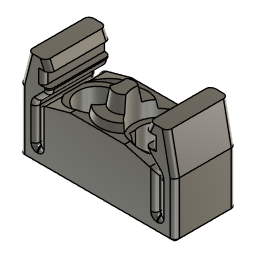
Lijn sensor lego adapter door Joep v9 (Autodesk Fusion 360 design; units mm, degrees)
Autodesk Fusion 360 part; units mm, degrees
note: some values were not read from the file. Chosen so that the rebuilt part matches the saved one: which face or edge a step refers to; which pieces of a blend or face edit are solid. Set by a fixed rule: which sketch regions a step uses.
sketch "Sketch1" plane through (0, 0, 0) normal (0, 1, 0) x (1, 0, 0)
  line L0 (41.5732, -34.0227) -> (56.5732, -34.0227)
  line L1 (41.5732, -34.0227) -> (41.5732, -28.0227)
  line L2 (41.5732, -28.0227) -> (41.0732, -28.0227)
  line L3 (42.0732, -35.2227) -> (42.0732, -37.0227)
  line L4 (42.0732, -37.0227) -> (42.8732, -37.0227)
  line L5 (42.8732, -37.0227) -> (42.3408, -38.2227)
  line L6 (42.3408, -38.2227) -> (39.0732, -38.2227)
  line L7 (49.0732, -34.0227) -> (49.0732, -26.0227) construction
  line L8 (42.8732, -34.6227) -> (41.0732, -32.8227)
  line L9 (41.0732, -32.8227) -> (41.0732, -28.0227)
  line L10 (39.0732, -26.0227) -> (39.0732, -38.2227)
  line L11 (55.2732, -37.0227) -> (55.8057, -38.2227)
  line L12 (56.0732, -37.0227) -> (55.2732, -37.0227)
  line L13 (56.0732, -35.2227) -> (56.0732, -37.0227)
  line L14 (55.8057, -38.2227) -> (59.0732, -38.2227)
  line L15 (59.0732, -26.0227) -> (39.0732, -26.0227)
  line L16 (59.0732, -26.0227) -> (59.0732, -38.2227)
  line L17 (57.0732, -32.8227) -> (57.0732, -28.0227)
  line L18 (56.5732, -28.0227) -> (57.0732, -28.0227)
  line L19 (56.5732, -34.0227) -> (56.5732, -28.0227)
  line L20 (42.0732, -35.2227) -> (42.8732, -35.2227)
  line L21 (42.8732, -35.2227) -> (42.8732, -34.6227)
  line L22 (56.0732, -35.2227) -> (55.2732, -35.2227)
  line L23 (55.2732, -35.2227) -> (55.2732, -34.6227)
  line L24 (55.2732, -34.6227) -> (57.0732, -32.8227)
  line L25 (41.0732, -28.0227) -> (39.0732, -28.0227)
  line L26 (57.0732, -28.0227) -> (59.0732, -28.0227)
  dimension "d3" = 3
  dimension "d5" = 1.2
  dimension "d6" = 0.8
  dimension "d15" = 1.8
  dimension "d16" = 0.5
  dimension "d17" = 2
  dimension "d18" = 14
  dimension "d19" = 8
  dimension "d20" = 15
  dimension "d21" = 20
  dimension "d67" = 0.6
  dimension "d68" = 0.8
  dimension "d85" = 45
  dimension "d86" = 2
  constraint horizontal L0
  constraint perpendicular L0 L1
  constraint perpendicular L1 L2
  constraint perpendicular L3 L4
  constraint horizontal L6
  constraint vertical L7
  constraint perpendicular L2 L9
  constraint coincident L6.end L10.end
  constraint symmetric L10.start L7 L15.start
  constraint symmetric L0.start L7 L0.end
  constraint symmetric L1.end L7 L18.start
  constraint symmetric L3.start L7 L13.start
  constraint symmetric L3.end L7 L12.start
  constraint symmetric L4.end L7 L11.start
  constraint symmetric L5.end L7 L11.end
  constraint symmetric L6.end L7 L14.end
  constraint symmetric L7 L2.end L17.end
  constraint symmetric L7 L8.end L17.start
  constraint symmetric L7 L6.end L14.end
  constraint coincident L0.end L19.start
  constraint coincident L10.start L15.end
  constraint midpoint L0 L7.start
  constraint midpoint L7.end L15
  constraint perpendicular L3 L20
  constraint perpendicular L20 L21
  constraint symmetric L7 L20.end L22.end
  constraint symmetric L7 L8.start L23.end
  constraint coincident L13.start L22.start
  constraint coincident L10 L25.end
  constraint perpendicular L10 L25
  constraint coincident L16 L26.end
  constraint perpendicular L16 L26
  constraint vertical L17
  measures "d3" distance of L0 L4
  measures "d5" distance of L4 L6
  measures "d6" distance of L3.end L4.end
  measures "d15" distance of L3.start L3.end
  measures "d16" distance of L1 L9
  measures "d17" distance of L9 L10
  measures "d18" distance of L3 L13
  measures "d19" distance of L0 L15
  measures "d20" distance of L1 L19
  measures "d21" distance of L10 L16
  measures "d67" distance of L20.end L8.start
  measures "d68" distance of L3.start L20.end
  measures "d85" angle of L8 L9
  measures "d86" distance of L2 L15
extrude "Extrude1" add sketch "Sketch1" along normal blind 7.9 contours L0 L1 L8 | L0 L1 L2 L8 L10 L15 L16 L18 L19 L24 L25 L26 | L0 L19 L24
sketch "Sketch2" plane through (0, 0, 26.0227) normal (0, 0, -1) x (1, 0, 0)
  circle A0 centre (45.0732, -3.95) radius 2.5
  circle A1 centre (53.0732, -3.95) radius 2.5
  line L0 (45.0732, -3.95) -> (53.0732, -3.95) construction
  line L1 (49.0732, 0) -> (49.0732, -7.9) construction
  circle A2 centre (49.0732, -3.45) radius 1.65
  circle A3 centre (49.0732, -3.45) radius 3
  line L2 (59.0732, 0) -> (39.0732, 0)
  line L3 (59.0732, -7.9) -> (39.0732, -7.9)
  circle A4 centre (53.0732, -3.95) radius 3.25
  circle A5 centre (45.0732, -3.95) radius 3.25
  dimension "d12" = 5
  dimension "d13" = 8
  dimension "d23" = 0.5
  dimension "d24" = 3.3
  dimension "d25" = 6
  dimension "d34" = 6.5
  constraint equal A0 A1
  constraint coincident A0.centre L0.start
  constraint coincident A1.centre L0.end
  constraint horizontal L0
  constraint midpoint L0 L1
  constraint midpoint L1.start L2
  constraint midpoint L1.end L3
  constraint concentric A1 A4
  constraint concentric A0 A5
  constraint equal A4 A5
  constraint coincident A2.centre A3.centre
  constraint coincident L1 A2.centre
  measures "d12" diameter of A0
  measures "d13" distance of A0.centre A1.centre
  measures "d23" distance of L0 A2.centre
  measures "d24" diameter of A2
  measures "d25" diameter of A3
  measures "d34" diameter of A4
extrude "Extrude3" add sketch "Sketch2" against normal blind 1 from surface at -8 contours A0 A2 | A0 A2 A5 | A0 A2 A3 | A0 A2 A3 A5 | A0 A2 A3 A5 | A2 A3 A4 A5 | A2 A4 A5 | A2 A3 A4 A5 | A1 A2 A3 A4 | A1 A2 A4 | A1 A2 A3 A4 | A1 A2 | A1 A2 A3
extrude "Extrude4" add sketch "Sketch2" against normal blind 2 draft -10 from surface at -9 contours A0 A2 | A0 A2 A5 | A2 A4 A5 | A1 A2 A4 | A1 A2
chamfer "Chamfer1" distance 0.2 distance2 1 1 edges at (46.2763, 4.5348, 34.0227) measured on face at (43.0732, 3.7833, 34.0227)
extrude "Extrude2" cut sketch "Sketch2" against normal blind 10.5 contours A0 A2 | A0 A2 A3 | A0 A3 | A1 A2 | A1 A2 A3 | A1 A3
extrude "Extrude5" cut sketch "Sketch2" against normal blind 1 contours A0 A2 | A0 A2 A5 | A0 A2 A3 | A0 A2 A3 A5 | A0 A2 A3 A5 | A0 A3 | A0 A3 A5 | A1 A2 A3 A4 | A1 A2 A4 | A1 A2 A3 A4 | A1 A3 A4 | A1 A2 | A1 A2 A3 | A1 A3
extrude "Extrude6" cut sketch "Sketch2" against normal blind 4 from surface at -7 contours A0 A2 | A0 A2 A5 | A0 A2 A3 | A0 A2 A3 A5 | A0 A2 A3 A5 | A0 A3 | A0 A3 A5 | A1 A2 A3 A4 | A1 A2 A4 | A1 A2 A3 A4 | A1 A3 A4 | A1 A2 | A1 A2 A3 | A1 A3
chamfer "Chamfer3" distance 4 distance2 1.1 1 edges at (56.5732, 3.95, 34.0227) measured on face at (47.8281, 7.6631, 34.0227)
chamfer "Chamfer3" distance 1.1 distance2 4 1 edges at (41.5732, 3.95, 34.0227) measured on face at (41.5732, 2.6333, 32.0227)
extrude "Extrude8" add sketch "Sketch1" along normal up to surface (7.9 mm away) contours L0 L1 L8 | L0 L1 L3 L4 L5 L6 L8 L9 L10 L20 L21 L25 | L0 L19 L24 | L0 L11 L12 L13 L14 L16 L17 L19 L22 L23 L24 L26
chamfer "Chamfer5" distance 0.4 distance2 0.4 2 edges at (50.7424, 4.854, 27.0227) (42.7424, 4.854, 27.0227) measured on face at (55.5701, 4.0746, 31.0227) measured on face at (47.5701, 4.0746, 31.0227)
ref_plane "WorkPlane1" through (49.0732, 3.95, 27.0227) normal (-1, 0, 0) x (0, 0, 1)
sketch "Sketch3" plane through (0, 0, 27.0227) normal (0, 0, -1) x (1, 0, 0)
  arc A0 (47.5001, -2.5611) -> (47.4946, -3.328) centre (48.9475, -2.9548) ccw
  arc A1 (46.8361, -2.1773) -> (47.5001, -2.5611) centre (47.8938, -1.1137) ccw
  line L0 (47.5001, -2.5611) -> (47.6937, -1.8493) construction
  line L1 (47.5001, -2.5611) -> (49.4203, -3.0835) construction
  line L2 (47.4946, -3.328) -> (46.8361, -2.1773)
  circle A2 centre (45.0732, -3.95) radius 3.25
  circle A3 centre (45.0732, -3.95) radius 2.9
  circle A4 centre (45.0732, -3.95) radius 2.5
  dimension "d60" = 1.5
  constraint equal A0 A1
  constraint tangent A0 L0
  constraint tangent A1 L1
  constraint perpendicular L0 L1
  constraint coincident A0.end A4
  constraint coincident A1.start A4
  constraint tangent A0 A4
  constraint tangent A1 A4
  measures "d60" radius of A1
extrude "Extrude7" cut sketch "Sketch3" against normal blind 7.8 contours A0 A1 A4 | L2 A4 picked at (47.2401, -2.8383)
mirror "Mirror1" about plane through (49.0732, 3.95, 27.0227) normal (-1, 0, 0) of "Extrude7"
chamfer "Chamfer6" distance 1 distance2 5 1 edges at (59.0732, 3.95, 38.2227) measured on face at (56.8949, 5.2667, 38.2227)
chamfer "Chamfer6" distance 4 distance2 1 1 edges at (39.0732, 3.95, 38.2227) measured on face at (39.0732, 5.2667, 30.0894)
fillet "Fillet2" radius 0.2 4 edges at (57.0732, 3.95, 28.0227) (56.5732, 3.95, 28.0227) (41.5732, 3.95, 28.0227) (41.0732, 3.95, 28.0227)
fillet "Fillet2" radius 0.6 35 edges at (41.3232, 7.9, 28.0227) (41.5732, 7.9, 30.4727) (41.0732, 7.9, 30.4227) (57.0732, 7.9, 30.4227) (56.8232, 7.9, 28.0227) (56.5732, 7.9, 30.4727) (56.8232, 0, 28.0227) (56.5732, 0, 30.4727) (57.0732, 0, 30.4227) (41.0732, 0, 30.4227) (41.5732, 0, 30.4727) (41.3232, 0, 28.0227) (41.9732, 7.9, 33.7227) (42.8732, 7.9, 34.9227) (42.607, 7.9, 37.6227) (39.5732, 7.9, 36.2227) (39.0732, 7.9, 30.1227) (39.0732, 0, 30.1227) (39.5732, 0, 36.2227) (42.607, 0, 37.6227) (42.0732, 0, 36.1227) (42.8732, 0, 34.9227) (41.9732, 0, 33.7227) (55.5395, 0, 37.6227) (58.5732, 0, 35.7227) (58.5732, 7.9, 35.7227) (55.5395, 7.9, 37.6227) (56.0732, 0, 36.1227) (56.1732, 0, 33.7227) (59.0732, 0, 29.6227) (59.0732, 7.9, 29.6227) (56.1732, 7.9, 33.7227) (55.2732, 7.9, 34.9227) (56.0732, 7.9, 36.1227) (55.2732, 0, 34.9227)
fillet "Fillet2" radius 1 4 edges at (55.2732, 3.95, 34.6227) (42.8732, 3.95, 34.6227) (41.0732, 3.95, 32.8227) (57.0732, 3.95, 32.8227)
fillet "Fillet3" radius 1 2 edges at (41.5732, 3.95, 32.9227) (56.5732, 3.95, 32.9227)
chamfer "Chamfer7" distance 0.4 angle 45 8 edges at (49.0732, 7.9, 26.0227) (39.249, 7.7243, 26.0227) (39.0732, 3.95, 26.0227) (39.249, 0.1757, 26.0227) (49.0732, 0, 26.0227) (58.8975, 0.1757, 26.0227) (59.0732, 3.95, 26.0227) (58.8975, 7.7243, 26.0227)
